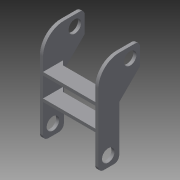
# Autodesk Inventor part: new_leg_1
Saved by Autodesk Inventor 2014 SP1 (Build 180222100, 222)
## iProperties
Created: 2014-12-05
Part Number: new_leg_1
Material: Générique
Document SubType Name: Modeling
Designer: astralien3000
Density: 1 g/cm^3
Appearance: Par défaut
d0: 50,000 mm
d1: 3,000 mm
d2: 3,000 mm
d3: 3,000 mm
d4: 3,000 mm
d5: 25,000 mm
d6: 90,000 mm
d7: 25,000 mm
d9: 45,000 mm
d10: 12,500 mm
d11: 40,000 mm
d12: 0,00 deg
d13: 7,000 mm
d14: 12,000 mm
d18: 0,00 deg
Author: astralien3000
Autodesk Inventor part; units mm, degrees
ref_plane "YZ Plane" through (0, 0, 0) normal (1, 0, 0) x (0, 1, 0)
ref_plane "XZ Plane" through (0, 0, 0) normal (0, 1, 0) x (-1, 0, 0)
ref_plane "XY Plane" through (0, 0, 0) normal (0, 0, 1) x (1, 0, 0)
sketch "Esquisse1" plane through (0, 0, 0) normal (0, 1, 0) x (-1, 0, 0)
  line L0 (-25, -45) -> (-28, -45)
  line L1 (-28, -45) -> (-28, 45)
  line L2 (-28, 45) -> (-25, 45)
  line L3 (-25, 45) -> (-25, -45)
  line L4 (25, 45) -> (28, 45)
  line L5 (28, 45) -> (28, -45)
  line L6 (28, -45) -> (25, -45)
  line L7 (25, -45) -> (25, 45)
  line L8 (-25, 12.5) -> (25, 12.5)
  line L9 (25, 12.5) -> (25, 9.5)
  line L10 (25, 9.5) -> (-25, 9.5)
  line L11 (-25, 9.5) -> (-25, 12.5)
  line L12 (-25, -9.5) -> (25, -9.5)
  line L13 (25, -9.5) -> (25, -12.5)
  line L14 (25, -12.5) -> (-25, -12.5)
  line L15 (-25, -12.5) -> (-25, -9.5)
  point P0 (0, 0)
  dimension "d0" = 50
  dimension "d1" = 3
  dimension "d2" = 3
  dimension "d3" = 3
  dimension "d4" = 3
  dimension "d5" = 25
  dimension "d6" = 90
  dimension "d7" = 25
  dimension "d9" = 45
  dimension "d10" = 12.5
  constraints: 32 end point, 8 parallel, 4 horizontal, 4 perpendicular, 4 point on line, 2 collinear
  measures "d0" distance between parallel lines of L7 L3
  measures "d1" distance between parallel lines of L5 L7
  measures "d2" distance between parallel lines of L3 L1
  measures "d3" distance between parallel lines of L10 L8
  measures "d4" distance between parallel lines of L12 L14
  measures "d5" distance from line of point (0, 0) L7
  measures "d6" distance between parallel lines of L4 L6
  measures "d7" distance between parallel lines of L14 L8
  measures "d9" distance from line of L6 point (0, 0)
  measures "d10" distance from line of point (0, 0) L14
extrude "Extrusion1" add sketch "Esquisse1" along normal blind 40 contours L0 L1 L2 L3 | L3 L12 L7 L14 | L7 L4 L5 L6 | L3 L8 L7 L10
sketch "Esquisse2" plane through (28, 0, 45) normal (1, 0, 0) x (0, 0, -1)
  line L0 (90, 0) -> (90, 40) projected
  line L1 (0, 0) -> (0, 40) projected
  circle A0 centre (80, 9.5) radius 6
  line L2 (0, 40) -> (90, 40) projected
  line L3 (80, 9.5) -> (10, 9.5) construction
  line L4 (10, 9.5) -> (10, 30.5) construction
  line L5 (10, 30.5) -> (80, 30.5) construction
  line L6 (80, 30.5) -> (80, 9.5) construction
  circle A1 centre (10, 30.5) radius 6
  line L7 (0, 0) -> (90, 0) projected
  line L8 (90, 40) -> (41, 40)
  line L9 (41, 40) -> (41, 20)
  line L10 (41, 20) -> (90, 20)
  line L11 (90, 20) -> (90, 40)
  line L12 (41, 40) -> (21, 40)
  line L13 (21, 40) -> (21, 20) construction
  line L14 (21, 20) -> (41, 20) construction
  line L15 (41, 20) -> (41, 40)
  line L16 (41, 20) -> (21, 40)
  point P0 (45, 0)
  dimension "d14" = 12
  dimension "d21" = 10
  dimension "d22" = 10
  dimension "d23" = 12
  dimension "d24" = 21
  dimension "d25" = 9.5
  dimension "d26" = 40
  dimension "d27" = 20
  dimension "d28" = 20
  dimension "d29" = 21
  constraints: 26 end point, 6 parallel, 3 horizontal, 3 perpendicular, 2 centre point, 2 point on line, 1 coincident, 1 collinear
  measures "d14" diameter of A0
  measures "d21" distance between parallel lines of L1 L4
  measures "d22" distance between parallel lines of L0 L6
  measures "d23" diameter of A1
  measures "d24" distance between parallel lines of L3 L5
  measures "d25" distance between parallel lines of L2 L5
  measures "d26" distance of L1.start L1.end
  measures "d27" distance between parallel lines of L7 L10
  measures "d28" distance between parallel lines of L9 L13
  measures "d29" distance between parallel lines of L1 L13
extrude "Extrusion2" cut sketch "Esquisse2" against normal through all contours L10 L9 L2 L0 | L16 L2 L9 | A0 | A1
sketch "Esquisse4" plane through (-25, 0, 12.5) normal (0, 0, 1) x (1, 0, 0)
  line L0 (50, 28.5) -> (0, 28.5) projected
  line L1 (0, 0) -> (0, 28.5) projected
  line L2 (0, 0) -> (50, 0) projected
  line L3 (0, 0) -> (50, 0)
  line L4 (50, 0) -> (50, 15)
  line L5 (50, 15) -> (0, 15)
  line L6 (0, 15) -> (0, 0)
  line L7 (50, 0) -> (50, 40) projected
  line L8 (50, 40) -> (53, 40) projected
  point P0 (25, 0)
  dimension "d33" = 25
  constraints: 8 end point, 2 parallel, 1 collinear, 1 horizontal, 1 perpendicular
  measures "d33" distance between parallel lines of L8 L5
extrude "Extrusion3" cut sketch "Esquisse4" against normal through all contours L7 L5 L1 L0
fillet "Congé2" radius 20 2 edges at (26.5, 0, 45) (-26.5, 0, 45)
fillet "Congé3" radius 5 6 edges at (26.5, 40, 45) (-26.5, 40, 45) (26.5, 20, -45) (26.5, 0, -45) (-26.5, 20, -45) (-26.5, 0, -45)
chamfer "Chanfrein1" distance 4 angle 45 4 edges at (-25, 15, 11) (-25, 15, -11) (25, 15, -11) (25, 15, 11)
equation "\"d2\" = d1"
equation "\"d4\" = d3"
equation "\"d5\" = 0.5 * d0"
equation "\"d9\" = 0.5 * d6"
equation "\"d10\" = 0.5 * d7"
equation "\"d23\" = d14"
equation "\"d25\" = -0.5 * d24 + 0.5 * d26"
equation "\"d27\" = 0.5 * d26"
equation "\"d28\" = d27"
